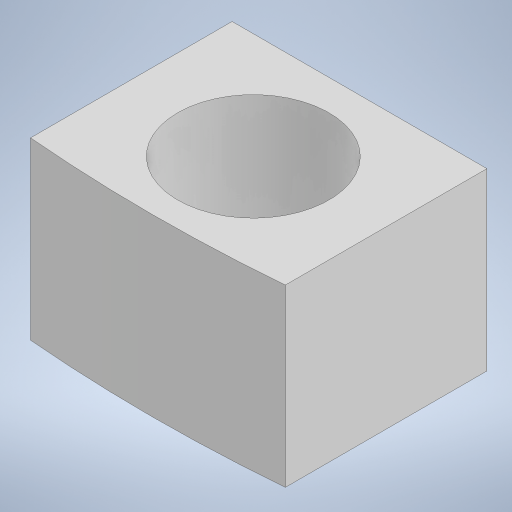
# Autodesk Inventor part: 100MagnetHolder
Saved by Autodesk Inventor 2024 (Build 280153000, 153)
## iProperties
Created: 2023-09-22
Part Number: 100MagnetHolder
Material: Generic
Document SubType Name: Modeling
Designer: Chris
Density: 1 g/cm^3
Appearance: Default
Author: Chris
Autodesk Inventor part; units mm, degrees
ref_plane "YZ Plane" through (0, 0, 0) normal (1, 0, 0) x (0, 1, 0)
ref_plane "XZ Plane" through (0, 0, 0) normal (0, 1, 0) x (-1, 0, 0)
ref_plane "XY Plane" through (0, 0, 0) normal (0, 0, 1) x (1, 0, 0)
sketch "Sketch1" plane through (0, 0, 0) normal (0, 1, 0) x (-1, 0, 0)
  circle A0 centre (0, 0) radius 50
  circle A1 centre (0, 0) radius 46.5
  circle A2 centre (0, 43.3342) radius 2.375
  line L0 (17.4744, 40) -> (-15.3474, 40)
  line L1 (4, 40) -> (4, 46.3276)
  line L2 (-4, 40) -> (-4, 46.3276)
  line L3 (0, 50) -> (0, 0)
  dimension "d0" = 100
  dimension "d1" = 93
  dimension "d2" = 4.75
  dimension "d6" = 40
  dimension "d8" = 4
  dimension "d10" = 4
  dimension "d11" = 4
  dimension "d12" = 0
  constraints: 8 end point, 2 centre point, 2 coincident, 2 point on circle, 2 point on line, 2 vertical, 1 horizontal, 1 parallel, 1 vertical alignment, 2 other
  measures "d1" diameter of A1
  measures "d2" diameter of A2
  measures "d6" distance from line of point (0, 0) L0
  measures "d8" distance between parallel lines of L1 L3
  measures "d10" distance from line of A2.centre L1
  measures "d11" distance from line of L2 A2.centre
  measures "d12" horizontal distance of point (0, 0) A2.centre
extrude "Extrusion1" add sketch "Sketch1" along normal blind 5.5 contours L1 L0 L3 A2 A1 | A1 L3 A2 L0 L2
body "Solid1"
